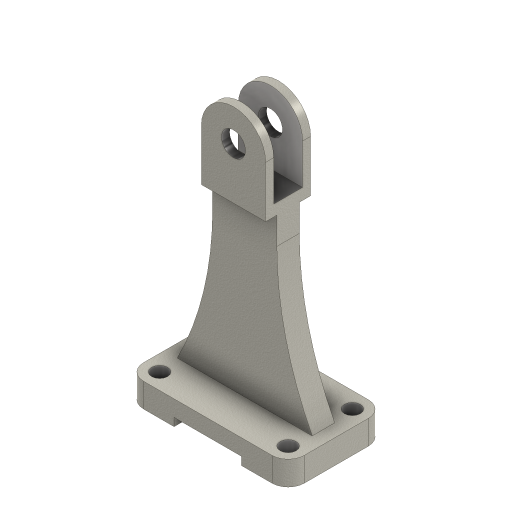
# Autodesk Inventor part: Part012. HighStand
Saved by Autodesk Inventor 2023.2 (Build 272271030, 271C)
## iProperties
Created: 2023-09-12
Part Number: Part012. HighStand
Material: Steel, Cast
Document SubType Name: Modeling
Designer: User
Mass: 1354.35 g
Surface Area: 406.446 cm^2
Volume: 172.528 cm^3
Density: 7.85 g/cm^3
Appearance: Steel - Cast
Author: User
Autodesk Inventor part; units mm, degrees
ref_plane "YZ Plane" through (0, 0, 0) normal (1, 0, 0) x (0, 1, 0)
ref_plane "XZ Plane" through (0, 0, 0) normal (0, 1, 0) x (-1, 0, 0)
ref_plane "XY Plane" through (0, 0, 0) normal (0, 0, 1) x (1, 0, 0)
sketch "Sketch1" plane through (0, 0, 0) normal (0, 1, 0) x (-1, 0, 0)
  line L0 (50, 30) -> (-50, 30)
  line L1 (-50, 30) -> (-50, -30)
  line L2 (-50, -30) -> (50, -30)
  line L3 (50, -30) -> (50, 30)
  line L4 (50, 30) -> (-50, -30) construction
  line L5 (-50, 30) -> (50, -30) construction
  point P0 (0, 0)
  dimension "d0" = 100
  dimension "d1" = 60
  constraints: 12 end point, 2 midpoint, 2 parallel, 1 horizontal, 1 perpendicular
  measures "d0" distance of L1.end L2.end
  measures "d1" distance of L0.end L1.end
extrude "Extrusion1" add sketch "Sketch1" along normal blind 15
fillet "Fillet1" radius 10 4 edges at (50, 7.5, -30) (-50, 7.5, -30) (-50, 7.5, 30) (50, 7.5, 30)
sketch "Sketch2" plane through (0, 0, 0) normal (0, 0, 1) x (1, 0, 0)
  line L0 (40, 0) -> (-40, 0) projected
  arc A0 (20, 155) -> (-20, 155) centre (0, 155) ccw
  line L1 (-20, 155) -> (-20, 106.1921)
  arc A1 (-42, 15) -> (-20, 106.1921) centre (-220, 106.1921) ccw
  line L2 (40, 15) -> (-40, 15) projected
  line L3 (0, 155) -> (0, -9.0216)
  line L4 (20, 155) -> (20, 106.1921)
  arc A2 (20, 106.1921) -> (42, 15) centre (220, 106.1921) ccw
  line L5 (-42, 15) -> (42, 15)
  line L6 (-50, 15) -> (-40, 15) projected
  point P0 (0, 0)
  point P1 (0, 0)
  dimension "d5" = 20
  dimension "d6" = 155
  dimension "d7" = 84
  dimension "d8" = 200
  constraints: 8 end point, 6 point on circle, 4 symmetric about line, 3 centre point, 2 vertical, 1 collinear, 1 midpoint, 1 point on line, 1 tangent, 1 vertical alignment, 1 other
  measures "d5" radius of A0
  measures "d6" distance of point (0, 0) L3.start
  measures "d7" distance of L5.end L5.start
  measures "d8" radius of A2
extrude "Extrusion2" add sketch "Sketch2" along normal mid plane 14
sketch "Sketch3" plane through (0, 0, 0) normal (0, 0, 1) x (1, 0, 0)
  line L0 (-20, 106.1921) -> (-20, 155) projected
  line L1 (-20, 123) -> (20, 123)
  line L2 (20, 155) -> (20, 106.1921) projected
  arc A0 (20, 155) -> (-20, 155) centre (0, 155) ccw projected
  line L3 (-20, 155) -> (-20, 123)
  line L4 (20, 123) -> (20, 155)
  point P0 (0, 0)
  dimension "d11" = 32
  constraints: 6 end point, 1 collinear, 1 horizontal, 1 point on line, 1 vertical
  measures "d11" distance from line of L1 A0.centre
extrude "Extrusion3" add sketch "Sketch3" along normal mid plane 28
sketch "Sketch4" plane through (20, 106.1921, 7) normal (1, 0, 0) x (0, 0, -1)
  line L0 (0, 0) -> (14, 0) projected
  line L1 (21, 48.8079) -> (-7, 48.8079) projected
  line L2 (-2, 68.8079) -> (16, 68.8079)
  line L3 (16, 68.8079) -> (16, 23.8079)
  line L4 (16, 23.8079) -> (-2, 23.8079)
  line L5 (-2, 23.8079) -> (-2, 68.8079)
  line L6 (21, 68.8079) -> (-7, 68.8079) projected
  point P0 (7, -106.1921)
  point P1 (7, 23.8079)
  point P2 (7, 0)
  dimension "d14" = 25
  dimension "d15" = 18
  constraints: 8 end point, 2 midpoint, 2 parallel, 1 collinear, 1 horizontal, 1 perpendicular, 1 vertical alignment
  measures "d14" distance between parallel lines of L4 L1
  measures "d15" distance between parallel lines of L3 L5
extrude "Extrusion4" cut sketch "Sketch4" against normal through all
sketch "Sketch5" plane through (-40, 0, 30) normal (0, 0, 1) x (1, 0, 0)
  line L0 (0, 0) -> (80, 0) projected
  line L1 (19, 5) -> (61, 5)
  line L2 (61, 5) -> (61, 0)
  line L3 (61, 0) -> (19, 0)
  line L4 (19, 0) -> (19, 5)
  point P0 (40, 0)
  point P1 (40, 0)
  point P2 (61, 0)
  dimension "d18" = 42
  dimension "d19" = 5
  constraints: 8 end point, 2 midpoint, 2 parallel, 1 horizontal, 1 perpendicular
  measures "d18" distance of L2.end L3.end
  measures "d19" distance between parallel lines of L0 L1
extrude "Extrusion5" cut sketch "Sketch5" against normal through all
sketch "Sketch6" plane through (0, 0, 14) normal (0, 0, 1) x (1, 0, 0)
  arc A0 (20, 155) -> (-20, 155) centre (0, 155) ccw projected
  point P0 (0, 0)
  constraints: 1 coincident
hole "Hole1" at (0, 155, 14) direction (0, 0, -1) diameter 15 end through all
sketch "Sketch7" plane through (0, 15, 0) normal (0, 1, 0) x (1, 0, 0)
  arc A0 (40, -30) -> (50, -20) centre (40, -20) ccw projected
  arc A1 (50, 20) -> (40, 30) centre (40, 20) ccw projected
  arc A2 (-40, 30) -> (-50, 20) centre (-40, 20) ccw projected
  arc A3 (-50, -20) -> (-40, -30) centre (-40, -20) ccw projected
  point P0 (0, 0)
hole "Hole2" at (-40, 15, -20) at (-40, 15, 20) at (40, 15, -20) at (40, 15, 20) direction (0, -1, 0) diameter 10 end through all
body "Solid1"
